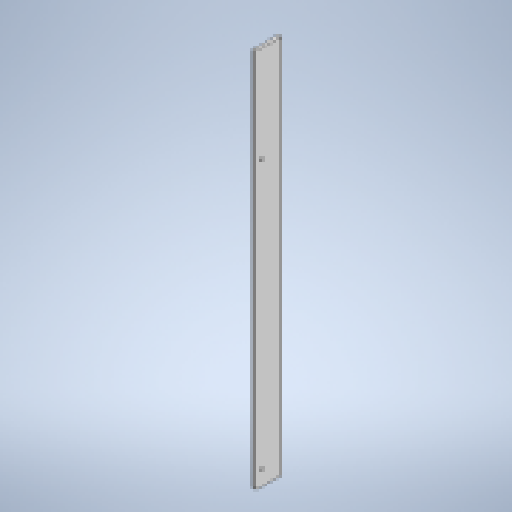
# Autodesk Inventor part: LBracket
Saved by Autodesk Inventor 2023 (Build 270158000, 158)
## iProperties
Created: 2022-09-10
Part Number: LBracket
Material: Generic
Document SubType Name: Modeling
Designer: deli
Density: 1 g/cm^3
Appearance: Default
Author: deli
Autodesk Inventor part; units mm, degrees
ref_plane "YZ Plane" through (0, 0, 0) normal (1, 0, 0) x (0, 1, 0)
ref_plane "XZ Plane" through (0, 0, 0) normal (0, 1, 0) x (-1, 0, 0)
ref_plane "XY Plane" through (0, 0, 0) normal (0, 0, 1) x (1, 0, 0)
sketch "Sketch1" plane through (0, 0, 0) normal (0, 1, 0) x (-1, 0, 0)
  line L0 (-3.8239, 51.1225) -> (-6.9989, 51.1225)
  line L1 (-6.9989, 51.1225) -> (-6.9989, 25.7225)
  line L2 (-6.9989, 25.7225) -> (18.4011, 25.7225)
  line L3 (18.4011, 25.7225) -> (18.4011, 28.8975)
  line L4 (18.4011, 28.8975) -> (-3.8239, 28.8975)
  line L5 (-3.8239, 28.8975) -> (-3.8239, 51.1225)
  point P0 (0, 0)
  dimension "d0" = 25.4
  dimension "d1" = 25.4
  dimension "d2" = 3.175
  dimension "d3" = 3.175
  constraints: 12 end point, 2 horizontal, 2 parallel, 2 perpendicular
  measures "d0" distance of L2.end L1.end
  measures "d1" distance of L1.end L0.end
  measures "d2" distance between parallel lines of L1 L5
  measures "d3" distance between parallel lines of L2 L4
extrude "Extrusion1" add sketch "Sketch1" along normal blind 300
sketch "Sketch2" plane through (6.9989, 0, 51.1225) normal (1, 0, 0) x (0, 0, -1)
  circle A0 centre (5.225, 15) radius 1.6 projected
  circle A1 centre (5.225, 285) radius 1.6 projected
  circle A2 centre (18.725, 37.7) radius 3.5
  line L0 (25.4, 0) -> (25.4, 300) projected
  line L1 (0, 0) -> (25.4, 0) projected
  line L2 (28.575, 50) -> (25.4, 50)
  point P0 (51.1225, 0)
  dimension "d18" = 7
  dimension "d19" = 6.675
  dimension "d20" = 37.7
  constraints: 2 end point, 1 centre point, 1 horizontal, 2 other
  measures "d18" diameter of A2
  measures "d19" distance from line of L0 A2.centre
  measures "d20" distance from line of L1 A2.centre
extrude "Extrusion2" cut sketch "Sketch2" against normal blind 10
sketch "Sketch3" plane through (-18.4011, 0, 28.8975) normal (0, 0, 1) x (1, 0, 0)
  circle A0 centre (11.1125, 8) radius 2
  circle A1 centre (11.1125, 292) radius 2
  point P0 (18.4011, 0)
  constraints: 2 centre point, 4 other
extrude "Extrusion3" cut sketch "Sketch3" against normal blind 10
sketch "Sketch4" plane through (0, 300, 0) normal (0, 1, 0) x (1, 0, 0)
  line L0 (6.9989, -51.1225) -> (6.9989, -25.7225) projected
  line L1 (6.9989, -25.7225) -> (-18.4011, -25.7225) projected
  line L2 (-18.4011, -25.7225) -> (-18.4011, -28.8975) projected
  line L3 (-18.4011, -28.8975) -> (3.8239, -28.8975) projected
  line L4 (3.8239, -28.8975) -> (3.8239, -51.1225) projected
  line L5 (3.8239, -51.1225) -> (6.9989, -51.1225) projected
  line L6 (3.8239, -28.8975) -> (3.8239, -25.7225)
  line L7 (3.8239, -43.1225) -> (6.9989, -43.1225)
  point P0 (0, 0)
  dimension "d12" = 8
  constraints: 4 end point, 3 point on line, 2 perpendicular
  measures "d12" distance between parallel lines of L7 L5
extrude "Extrusion4" add sketch "Sketch4" along normal blind 82.6 contours L5 L4 L7 L0
fillet "Fillet1" radius 4 1 edges at (5.4114, 300, 43.1225)
sketch "Sketch5" plane through (6.9989, 0, 51.1225) normal (1, 0, 0) x (0, 0, -1)
  circle A0 centre (4, 378.6) radius 2
  circle A1 centre (4, 378.6) radius 4
  line L0 (0, 382.6) -> (8, 382.6) projected
  line L1 (0, 0) -> (0, 382.6) projected
  line L2 (8, 304) -> (8, 382.6) projected
  point P0 (51.1225, 0)
  point P1 (0, 378.6)
  point P2 (4, 382.6)
  point P3 (8, 378.6)
  dimension "d14" = 4
  dimension "d15" = 8
  constraints: 2 centre point, 2 tangent, 1 coincident
  measures "d14" diameter of A0
  measures "d15" diameter of A1
extrude "Extrusion5" cut sketch "Sketch5" against normal blind 82.6 contours A0 | A1 L0 L2 | A1 L1 L0
body "Solid1"
